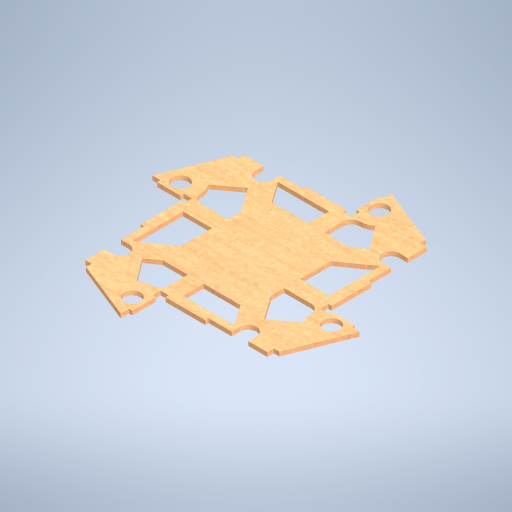
# Autodesk Inventor part: plate
Saved by Autodesk Inventor 2024.1 (Build 281209000, 209)
## iProperties
Created: 2024-07-03
Part Number: plate
Material: 木材 (サクラ材)
Document SubType Name: Modeling
Designer: hibik
Density: 0.63 g/cm^3
Appearance: サクラ材 - ナチュラル 抑えた光沢
Author: hibik
Autodesk Inventor part; units mm, degrees
ref_plane "YZ Plane" through (0, 0, 0) normal (1, 0, 0) x (0, 1, 0)
ref_plane "XZ Plane" through (0, 0, 0) normal (0, 1, 0) x (-1, 0, 0)
ref_plane "XY Plane" through (0, 0, 0) normal (0, 0, 1) x (1, 0, 0)
sketch "スケッチ1" plane through (0, 0, 0) normal (0, 1, 0) x (-1, 0, 0)
  line L0 (26.5, 31.5) -> (-26.5, 31.5)
  line L1 (-26.5, 31.5) -> (-26.5, -31.5)
  line L2 (-26.5, -31.5) -> (26.5, -31.5)
  line L3 (26.5, -31.5) -> (26.5, 31.5)
  line L4 (26.5, 31.5) -> (-26.5, -31.5) construction
  line L5 (-26.5, 31.5) -> (26.5, -31.5) construction
  point P0 (0, 0)
  dimension "d0" = 53
  dimension "d1" = 63
  constraints: 12 end point, 2 midpoint, 2 parallel, 1 horizontal, 1 perpendicular
  measures "d0" distance of L2.end L1.end
  measures "d1" distance of L1.end L0.end
extrude "押し出し1" add sketch "スケッチ1" along normal blind 2.5
sketch "スケッチ6" plane through (0, 0, 0) normal (0, -1, 0) x (1, 0, 0)
  arc A0 (26.3287, -65.2977) -> (29.0118, -58.5429) centre (24.4787, -60.6525) ccw projected
  line L0 (26.3287, -65.2977) -> (44.15, -58.2) projected
  line L1 (44.15, -54.8) -> (44.15, -58.2) projected
  line L2 (46.15, -54.8) -> (44.15, -54.8) projected
  line L3 (46.15, -54.8) -> (48, -54.8) projected
  line L4 (48, -43.3721) -> (48, -54.8) projected
  line L5 (48, -43.3721) -> (43, -43.3721) projected
  arc A1 (40.1241, -42.4623) -> (43, -43.3721) centre (43, -38.3721) ccw projected
  line L6 (40.1241, -42.4623) -> (42.3111, -44) projected
  arc A2 (36.5717, -56.5915) -> (42.3111, -44) centre (32.8717, -47.3012) ccw projected
  line L7 (36.5717, -56.5915) -> (32.1435, -58.3551) projected
  arc A3 (29.0118, -58.5429) -> (32.1435, -58.3551) centre (30.2935, -53.7099) ccw projected
  line L8 (-26.5, 18.6328) -> (-26.5, 0) projected
  line L9 (-26.5, 0) -> (-44, 0) projected
  line L10 (-44, 0) -> (-44, 30.9375) projected
  line L11 (-44, 30.9375) -> (-26.5, 18.6328) projected
  line L12 (22.5, 27.5) -> (22.5, -27.5) projected
  line L13 (22.5, -27.5) -> (-22.5, -27.5) projected
  line L14 (-22.5, -27.5) -> (-22.5, 27.5) projected
  line L15 (-22.5, 27.5) -> (22.5, 27.5) projected
  line L16 (22.1484, 31.5) -> (0, 31.5) projected
  line L17 (0, 31.5) -> (0, 44) projected
  line L18 (0, 44) -> (30.9375, 44) projected
  line L19 (30.9375, 44) -> (22.1484, 31.5) projected
  line L20 (26.5, -18.6328) -> (26.5, 0) projected
  line L21 (26.5, 0) -> (44, 0) projected
  line L22 (44, 0) -> (44, -30.9375) projected
  line L23 (44, -30.9375) -> (26.5, -18.6328) projected
  line L24 (-22.1484, -31.5) -> (0, -31.5) projected
  line L25 (0, -31.5) -> (0, -44) projected
  line L26 (0, -44) -> (-30.9375, -44) projected
  line L27 (-30.9375, -44) -> (-22.1484, -31.5) projected
  arc A4 (25.7604, -55.8196) -> (19.4893, -60.3263) centre (24.4787, -60.6525) ccw projected
  arc A5 (25.6484, -55.56) -> (25.7604, -55.8196) centre (30.2935, -53.7099) ccw projected
  arc A6 (25.6484, -55.56) -> (14.5, -48) centre (14.5, -60) ccw projected
  arc A7 (9.5, -43) -> (14.5, -48) centre (14.5, -43) ccw projected
  line L28 (9.5, -43) -> (9.5, -31.5) projected
  line L29 (9.5, -31.5) -> (24.5333, -31.5) projected
  line L30 (24.5333, -31.5) -> (40.1241, -42.4623) projected
  arc A8 (39.1622, -35.1673) -> (40.1241, -42.4623) centre (43, -38.3721) ccw projected
  circle A9 centre (35.3243, -31.9624) radius 5 projected
  arc A10 (43, -33.3721) -> (39.1622, -35.1673) centre (43, -38.3721) ccw projected
  line L31 (43, -33.3721) -> (48, -33.3721) projected
  line L32 (48, -19.5) -> (48, -33.3721) projected
  line L33 (50, -19.5) -> (48, -19.5) projected
  line L34 (50, -19.5) -> (50, 4.5) projected
  line L35 (48, 4.5) -> (50, 4.5) projected
  line L36 (48, 9.5) -> (48, 4.5) projected
  line L37 (53, 9.5) -> (48, 9.5) projected
  line L38 (53, 7.5) -> (53, 9.5) projected
  line L39 (53, 7.5) -> (67, 7.5) projected
  line L40 (67, 9.5) -> (67, 7.5) projected
  line L41 (72, 9.5) -> (67, 9.5) projected
  line L42 (72, 9.5) -> (65.2977, 26.3287) projected
  arc A11 (60.3263, 19.4893) -> (65.2977, 26.3287) centre (60.6525, 24.4787) ccw projected
  circle A12 centre (60, 14.5) radius 5 projected
  arc A13 (55.8196, 25.7604) -> (60.3263, 19.4893) centre (60.6525, 24.4787) ccw projected
  arc A14 (55.56, 25.6484) -> (55.8196, 25.7604) centre (53.7099, 30.2935) ccw projected
  arc A15 (55.56, 25.6484) -> (48, 14.5) centre (60, 14.5) ccw projected
  arc A16 (43, 9.5) -> (48, 14.5) centre (43, 14.5) ccw projected
  line L43 (43, 9.5) -> (26.5, 9.5) projected
  line L44 (26.5, 9.5) -> (26.5, 17.4222) projected
  line L45 (26.5, 17.4222) -> (42.4623, 40.1241) projected
  arc A17 (35.1673, 39.1622) -> (42.4623, 40.1241) centre (38.3721, 43) ccw projected
  circle A18 centre (31.9624, 35.3243) radius 5 projected
  arc A19 (33.3721, 43) -> (35.1673, 39.1622) centre (38.3721, 43) ccw projected
  line L46 (33.3721, 43) -> (33.3721, 48) projected
  line L47 (19.5, 48) -> (33.3721, 48) projected
  line L48 (19.5, 50) -> (19.5, 48) projected
  line L49 (19.5, 50) -> (-4.5, 50) projected
  line L50 (-4.5, 48) -> (-4.5, 50) projected
  line L51 (-9.5, 48) -> (-4.5, 48) projected
  line L52 (-9.5, 53) -> (-9.5, 48) projected
  line L53 (-7.5, 53) -> (-9.5, 53) projected
  line L54 (-7.5, 53) -> (-7.5, 67) projected
  line L55 (-9.5, 67) -> (-7.5, 67) projected
  line L56 (-9.5, 72) -> (-9.5, 67) projected
  line L57 (-9.5, 72) -> (-26.3287, 65.2977) projected
  arc A20 (-19.4893, 60.3263) -> (-26.3287, 65.2977) centre (-24.4787, 60.6525) ccw projected
  circle A21 centre (-14.5, 60) radius 5 projected
  arc A22 (-25.7604, 55.8196) -> (-19.4893, 60.3263) centre (-24.4787, 60.6525) ccw projected
  arc A23 (-25.6484, 55.56) -> (-25.7604, 55.8196) centre (-30.2935, 53.7099) ccw projected
  arc A24 (-25.6484, 55.56) -> (-14.5, 48) centre (-14.5, 60) ccw projected
  arc A25 (-9.5, 43) -> (-14.5, 48) centre (-14.5, 43) ccw projected
  line L58 (-9.5, 43) -> (-9.5, 31.5) projected
  line L59 (-9.5, 31.5) -> (-24.5333, 31.5) projected
  line L60 (-24.5333, 31.5) -> (-40.1241, 42.4623) projected
  arc A26 (-39.1622, 35.1673) -> (-40.1241, 42.4623) centre (-43, 38.3721) ccw projected
  circle A27 centre (-35.3243, 31.9624) radius 5 projected
  arc A28 (-43, 33.3721) -> (-39.1622, 35.1673) centre (-43, 38.3721) ccw projected
  line L61 (-43, 33.3721) -> (-48, 33.3721) projected
  line L62 (-48, 19.5) -> (-48, 33.3721) projected
  line L63 (-50, 19.5) -> (-48, 19.5) projected
  line L64 (-50, 19.5) -> (-50, -4.5) projected
  line L65 (-48, -4.5) -> (-50, -4.5) projected
  line L66 (-48, -9.5) -> (-48, -4.5) projected
  line L67 (-53, -9.5) -> (-48, -9.5) projected
  line L68 (-53, -7.5) -> (-53, -9.5) projected
  line L69 (-53, -7.5) -> (-67, -7.5) projected
  line L70 (-67, -9.5) -> (-67, -7.5) projected
  line L71 (-72, -9.5) -> (-67, -9.5) projected
  line L72 (-72, -9.5) -> (-65.2977, -26.3287) projected
  arc A29 (-60.3263, -19.4893) -> (-65.2977, -26.3287) centre (-60.6525, -24.4787) ccw projected
  circle A30 centre (-60, -14.5) radius 5 projected
  arc A31 (-55.8196, -25.7604) -> (-60.3263, -19.4893) centre (-60.6525, -24.4787) ccw projected
  arc A32 (-55.56, -25.6484) -> (-55.8196, -25.7604) centre (-53.7099, -30.2935) ccw projected
  arc A33 (-55.56, -25.6484) -> (-48, -14.5) centre (-60, -14.5) ccw projected
  arc A34 (-43, -9.5) -> (-48, -14.5) centre (-43, -14.5) ccw projected
  line L73 (-43, -9.5) -> (-26.5, -9.5) projected
  line L74 (-26.5, -9.5) -> (-26.5, -17.4222) projected
  line L75 (-26.5, -17.4222) -> (-42.4623, -40.1241) projected
  arc A35 (-35.1673, -39.1622) -> (-42.4623, -40.1241) centre (-38.3721, -43) ccw projected
  circle A36 centre (-31.9624, -35.3243) radius 5 projected
  arc A37 (-33.3721, -43) -> (-35.1673, -39.1622) centre (-38.3721, -43) ccw projected
  line L76 (-33.3721, -43) -> (-33.3721, -48) projected
  line L77 (-19.5, -48) -> (-33.3721, -48) projected
  line L78 (-19.5, -50) -> (-19.5, -48) projected
  line L79 (-19.5, -50) -> (4.5, -50) projected
  line L80 (4.5, -48) -> (4.5, -50) projected
  line L81 (9.5, -48) -> (4.5, -48) projected
  line L82 (9.5, -53) -> (9.5, -48) projected
  line L83 (7.5, -53) -> (9.5, -53) projected
  line L84 (7.5, -53) -> (7.5, -67) projected
  line L85 (9.5, -67) -> (7.5, -67) projected
  line L86 (9.5, -72) -> (9.5, -67) projected
  line L87 (9.5, -72) -> (26.3287, -65.2977) projected
  arc A38 (19.4893, -60.3263) -> (26.3287, -65.2977) centre (24.4787, -60.6525) ccw projected
  circle A39 centre (14.5, -60) radius 5 projected
  arc A40 (-65.2977, -26.3287) -> (-58.5429, -29.0118) centre (-60.6525, -24.4787) ccw projected
  line L88 (-65.2977, -26.3287) -> (-58.2, -44.15) projected
  line L89 (-54.8, -44.15) -> (-58.2, -44.15) projected
  line L90 (-54.8, -46.15) -> (-54.8, -44.15) projected
  line L91 (-54.8, -46.15) -> (-54.8, -48) projected
  line L92 (-43.3721, -48) -> (-54.8, -48) projected
  line L93 (-43.3721, -48) -> (-43.3721, -43) projected
  arc A41 (-42.4623, -40.1241) -> (-43.3721, -43) centre (-38.3721, -43) ccw projected
  line L94 (-42.4623, -40.1241) -> (-44, -42.3111) projected
  arc A42 (-56.5915, -36.5717) -> (-44, -42.3111) centre (-47.3012, -32.8717) ccw projected
  line L95 (-56.5915, -36.5717) -> (-58.3551, -32.1435) projected
  arc A43 (-58.5429, -29.0118) -> (-58.3551, -32.1435) centre (-53.7099, -30.2935) ccw projected
  arc A44 (-26.3287, 65.2977) -> (-29.0118, 58.5429) centre (-24.4787, 60.6525) ccw projected
  line L96 (-26.3287, 65.2977) -> (-44.15, 58.2) projected
  line L97 (-44.15, 54.8) -> (-44.15, 58.2) projected
  line L98 (-46.15, 54.8) -> (-44.15, 54.8) projected
  line L99 (-46.15, 54.8) -> (-48, 54.8) projected
  line L100 (-48, 43.3721) -> (-48, 54.8) projected
  line L101 (-48, 43.3721) -> (-43, 43.3721) projected
  arc A45 (-40.1241, 42.4623) -> (-43, 43.3721) centre (-43, 38.3721) ccw projected
  line L102 (-40.1241, 42.4623) -> (-42.3111, 44) projected
  arc A46 (-36.5717, 56.5915) -> (-42.3111, 44) centre (-32.8717, 47.3012) ccw projected
  line L103 (-36.5717, 56.5915) -> (-32.1435, 58.3551) projected
  arc A47 (-29.0118, 58.5429) -> (-32.1435, 58.3551) centre (-30.2935, 53.7099) ccw projected
  arc A48 (65.2977, 26.3287) -> (58.5429, 29.0118) centre (60.6525, 24.4787) ccw projected
  line L104 (65.2977, 26.3287) -> (58.2, 44.15) projected
  line L105 (54.8, 44.15) -> (58.2, 44.15) projected
  line L106 (54.8, 46.15) -> (54.8, 44.15) projected
  line L107 (54.8, 46.15) -> (54.8, 48) projected
  line L108 (43.3721, 48) -> (54.8, 48) projected
  line L109 (43.3721, 48) -> (43.3721, 43) projected
  arc A49 (42.4623, 40.1241) -> (43.3721, 43) centre (38.3721, 43) ccw projected
  line L110 (42.4623, 40.1241) -> (44, 42.3111) projected
  arc A50 (56.5915, 36.5717) -> (44, 42.3111) centre (47.3012, 32.8717) ccw projected
  line L111 (56.5915, 36.5717) -> (58.3551, 32.1435) projected
  arc A51 (58.5429, 29.0118) -> (58.3551, 32.1435) centre (53.7099, 30.2935) ccw projected
  line L112 (35.3243, -31.9624) -> (14.5, -60)
  line L113 (-31.9624, -35.3243) -> (-60, -14.5)
  line L114 (-35.3243, 31.9624) -> (-14.5, 60)
  line L115 (60, 14.5) -> (31.9624, 35.3243)
  point P0 (0, 0)
  point P1 (31.8479, -36.6431)
  point P2 (21.6551, -50.3665)
  point P3 (36.6431, 31.8479)
  point P4 (50.3665, 21.6551)
  point P5 (-31.8479, 36.6431)
  point P6 (-21.6551, 50.3665)
  point P7 (-36.6431, -31.8479)
  point P8 (-50.3665, -21.6551)
  constraints: 8 end point, 8 other
extrude "押し出し6" add sketch "スケッチ6" against normal blind 2.5 contours A38 A4 A5 A6 L112 L30 L6 A2 L7 A3 A0 | A0 A3 L7 A2 L6 A1 L5 L4 L3 L2 L1 L0 | L87 L86 L85 L84 L83 L82 L81 L80 L79 L78 L77 L76 A37 A36 L113 L75 L74 L73 A34 A33 A30 A29 L72 L71 L70 L69 L68 L67 L66 L65 L64 L63 L62 L61 A28 A27 L114 L60 L59 L58 A25 A24 A21 A20 L57 L56 L55 L54 L53 L52 L51 L50 L49 L48 L47 L46 A19 A18 L115 L45 L44 L43 A16 A15 A12 A11 L42 L41 L40 L39 L38 L37 L36 L35 L34 L33 L32 L31 A10 A9 L112 L30 L29 L28 A7 A6 A39 A38 | A39 L112 A6 A5 A4 | L112 A9 A8 L30 | A9 | A36 | A35 L75 L113 A36 | L94 A42 L95 A43 A40 A29 A31 A32 A33 L113 L75 | A41 L93 L92 L91 L90 L89 L88 A40 A43 L95 A42 L94 | A33 A32 A31 A30 L113 | A11 A13 A14 A15 L115 L45 L110 A50 L111 A51 A48 | A48 A51 L111 A50 L110 A49 L109 L108 L107 L106 L105 L104 | A12 L115 A15 A14 A13 | L115 A18 A17 L45 | A18 | A27 | A26 L60 L114 A27 | L102 A46 L103 A47 A44 A20 A22 A23 A24 L114 L60 | A45 L101 L100 L99 L98 L97 L96 A44 A47 L103 A46 L102 | A24 A23 A22 A21 L114
